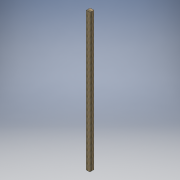
# Autodesk Inventor part: BedPost
Saved by Autodesk Inventor 2017 (Build 210142000, 142)
## iProperties
Created: 2016-10-24
Part Number: BedPost
Material: Generic
Document SubType Name: Modeling
Designer: andrew
Density: 1 g/cm^3
Appearance: Driftwood
Author: andrew
Autodesk Inventor part; units mm, degrees
ref_plane "YZ Plane" through (0, 0, 0) normal (1, 0, 0) x (0, 1, 0)
ref_plane "XZ Plane" through (0, 0, 0) normal (0, 1, 0) x (-1, 0, 0)
ref_plane "XY Plane" through (0, 0, 0) normal (0, 0, 1) x (1, 0, 0)
sketch "Sketch1" plane through (0, 0, 0) normal (0, 1, 0) x (-1, 0, 0)
  line L0 (-28.575, 31.75) -> (28.575, 31.75)
  line L1 (28.575, 31.75) -> (28.575, -31.75)
  line L2 (28.575, -31.75) -> (-28.575, -31.75)
  line L3 (-28.575, -31.75) -> (-28.575, 31.75)
  line L4 (-28.575, 31.75) -> (28.575, -31.75) construction
  line L5 (28.575, 31.75) -> (-28.575, -31.75) construction
  point P0 (0, 0)
  dimension "d0" = 63.5
  dimension "d1" = 57.15
  constraints: 12 end point, 2 midpoint, 2 parallel, 1 horizontal, 1 perpendicular
  measures "d0" distance of L0.end L1.end
  measures "d1" distance of L1.end L2.end
extrude "Extrusion1" add sketch "Sketch1" along normal blind 2133.6
body "Solid1"
